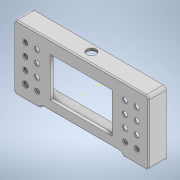
# Autodesk Inventor part: CONTROL_BOARD
Saved by Autodesk Inventor 2020 (Build 240168000, 168)
## iProperties
Created: 2020-06-05
Part Number: CONTROL_BOARD
Material: Generic
Document SubType Name: Modeling
Designer: Gebruiker
Density: 1 g/cm^3
Appearance: Default
Author: Gebruiker
Autodesk Inventor part; units mm, degrees
ref_plane "YZ Plane" through (0, 0, 0) normal (1, 0, 0) x (0, 1, 0)
ref_plane "XZ Plane" through (0, 0, 0) normal (0, 1, 0) x (-1, 0, 0)
ref_plane "XY Plane" through (0, 0, 0) normal (0, 0, 1) x (1, 0, 0)
sketch "Sketch1" plane through (0, 0, 0) normal (0, 0, 1) x (1, 0, 0)
  line L0 (-92.5, -50) -> (92.5, -50)
  line L1 (92.5, -50) -> (92.5, 50)
  line L2 (92.5, 50) -> (-92.5, 50)
  line L3 (-92.5, 50) -> (-92.5, -50)
  line L4 (-92.5, -50) -> (92.5, 50) construction
  line L5 (92.5, -50) -> (-92.5, 50) construction
  line L6 (70, 55) -> (115, 55)
  line L7 (115, 55) -> (115, 45)
  line L8 (115, 45) -> (70, 45)
  line L9 (70, 45) -> (70, 55)
  line L10 (70, 55) -> (115, 45) construction
  line L11 (115, 55) -> (70, 45) construction
  line L12 (70, -45) -> (115, -45)
  line L13 (115, -45) -> (115, -55)
  line L14 (115, -55) -> (70, -55)
  line L15 (70, -55) -> (70, -45)
  line L16 (70, -45) -> (115, -55) construction
  line L17 (115, -45) -> (70, -55) construction
  line L18 (-115, -45) -> (-70, -45)
  line L19 (-70, -45) -> (-70, -55)
  line L20 (-70, -55) -> (-115, -55)
  line L21 (-115, -55) -> (-115, -45)
  line L22 (-115, -45) -> (-70, -55) construction
  line L23 (-70, -45) -> (-115, -55) construction
  line L24 (-115, 55) -> (-70, 55)
  line L25 (-70, 55) -> (-70, 45)
  line L26 (-70, 45) -> (-115, 45)
  line L27 (-115, 45) -> (-115, 55)
  line L28 (-115, 55) -> (-70, 45) construction
  line L29 (-70, 55) -> (-115, 45) construction
  line L30 (70, 45) -> (115, 45)
  line L31 (115, 45) -> (115, -45)
  line L32 (115, -45) -> (70, -45)
  line L33 (70, -45) -> (70, 45)
  line L34 (70, 45) -> (115, -45) construction
  line L35 (115, 45) -> (70, -45) construction
  line L36 (-115, 45) -> (-70, 45)
  line L37 (-70, 45) -> (-70, -45)
  line L38 (-70, -45) -> (-115, -45)
  line L39 (-115, -45) -> (-115, 45)
  line L40 (-115, 45) -> (-70, -45) construction
  line L41 (-70, 45) -> (-115, -45) construction
  line L42 (115, 45) -> (115, 25)
  line L43 (115, -45) -> (115, -25)
  line L44 (-115, -45) -> (-115, -25)
  line L45 (-115, 45) -> (-115, 25)
  line L46 (-70, 55) -> (70, 55)
  line L47 (70, 55) -> (70, 50)
  line L48 (70, 50) -> (-70, 50)
  line L49 (-70, 50) -> (-70, 55)
  point P0 (0, 0)
  point P1 (92.5, 0)
  point P2 (-92.5, 0)
  point P3 (-70, -50)
  point P4 (70, -50)
  dimension "d0" = 185
  dimension "d1" = 100
  dimension "d2" = 45
  dimension "d3" = 10
  dimension "d4" = 45
  dimension "d5" = 10
  dimension "d6" = 45
  dimension "d7" = 45
  dimension "d8" = 10
  dimension "d9" = 45
  dimension "d10" = 90
  dimension "d20" = 20
  dimension "d21" = 20
  dimension "d22" = 20
  dimension "d23" = 20
  dimension "d83" = 45
  constraints: 100 end point, 17 midpoint, 16 parallel, 8 horizontal, 8 perpendicular, 6 point on line, 1 collinear
  measures "d0" distance of L2.end L1.end
  measures "d1" distance of L1.end L0.end
  measures "d2" distance of L7.end L8.end
  measures "d3" distance of L6.end L7.end
  measures "d4" distance of L13.end L14.end
  measures "d5" distance of L12.end L13.end
  measures "d6" distance of L19.end L20.end
  measures "d7" distance of L25.end L26.end
  measures "d8" distance of L24.end L25.end
  measures "d9" distance of L31.end L32.end
  measures "d10" distance of L36.end L37.end
  measures "d20" distance of L7.end L42.end
  measures "d21" distance of L12.end L43.end
  measures "d22" distance of L18.start L44.end
  measures "d23" distance of L26.end L45.end
  measures "d83" distance of L37.end L38.end
extrude "Extrusion1" add sketch "Sketch1" against normal blind 30
fillet "Fillet1" radius 5 8 edges at (-115, 55, -15) (-115, -55, -15) (-70, -55, -15) (-70, -50, -15) (70, -50, -15) (70, -55, -15) (115, -55, -15) (115, 55, -15)
sketch "Sketch5" plane through (0, 0, -30) normal (0, 0, -1) x (-1, 0, 0)
  line L0 (-109, 44) -> (109, 44)
  line L1 (109, 44) -> (109, -44)
  line L2 (109, -44) -> (-109, -44)
  line L3 (-109, -44) -> (-109, 44)
  line L4 (-109, 44) -> (109, -44) construction
  line L5 (109, 44) -> (-109, -44) construction
  point P0 (0, 0)
  dimension "d51" = 218
  dimension "d52" = 88
  constraints: 12 end point, 2 midpoint, 2 parallel, 1 horizontal, 1 perpendicular
  measures "d51" distance of L1.end L2.end
  measures "d52" distance of L0.end L1.end
extrude "Extrusion5" cut sketch "Sketch5" against normal blind 25
sketch "Sketch6" plane through (0, 0, 0) normal (0, 0, 1) x (1, 0, 0)
  line L0 (-53, 34) -> (53, 34)
  line L1 (53, 34) -> (53, -34)
  line L2 (53, -34) -> (-53, -34)
  line L3 (-53, -34) -> (-53, 34)
  line L4 (-53, 34) -> (53, -34) construction
  line L5 (53, 34) -> (-53, -34) construction
  point P0 (0, 0)
  dimension "d56" = 106
  dimension "d57" = 68
  constraints: 12 end point, 2 midpoint, 2 parallel, 1 horizontal, 1 perpendicular
  measures "d56" distance of L1.end L2.end
  measures "d57" distance of L0.end L1.end
extrude "Extrusion6" cut sketch "Sketch6" against normal blind 5
sketch "Sketch7" plane through (0, 0, 0) normal (0, 0, 1) x (1, 0, 0)
  line L0 (-53, -34) -> (-53, 34) projected
  line L1 (-53, 34) -> (53, 34) projected
  line L2 (53, 34) -> (53, -34) projected
  line L3 (53, -34) -> (-53, -34) projected
  arc A0 (-110, 55) -> (-115, 50) centre (-110, 50) ccw projected
  arc A1 (-115, -50) -> (-110, -55) centre (-110, -50) ccw projected
  line L4 (-110, -55) -> (-73.6603, -55) projected
  arc A2 (-73.6603, -55) -> (-69.3301, -52.5) centre (-73.6603, -50) ccw projected
  arc A3 (-65, -50) -> (-69.3301, -52.5) centre (-65, -55) ccw projected
  line L5 (-65, -50) -> (65, -50) projected
  arc A4 (69.3301, -52.5) -> (65, -50) centre (65, -55) ccw projected
  arc A5 (69.3301, -52.5) -> (73.6603, -55) centre (73.6603, -50) ccw projected
  line L6 (73.6603, -55) -> (110, -55) projected
  arc A6 (110, -55) -> (115, -50) centre (110, -50) ccw projected
  arc A7 (115, 50) -> (110, 55) centre (110, 50) ccw projected
  line L7 (110, 55) -> (-110, 55) projected
  line L8 (4.825, 59.0166) -> (4.825, -53.5355) construction
  line L9 (-115, 50) -> (-115, -50) projected
  line L10 (115, -50) -> (115, 50) projected
  point P0 (0, 0)
  constraints: 2 end point, 1 vertical
sketch "Sketch8" plane through (0, 0, 0) normal (0, 0, 1) x (1, 0, 0)
  line L0 (67.7, 39.3) -> (83, 39.3)
  line L1 (83, 39.3) -> (83, 24.3)
  line L2 (83, 24.3) -> (67.7, 24.3)
  line L3 (67.7, 24.3) -> (67.7, 39.3)
  line L4 (87.7, 39.3) -> (103, 39.3)
  line L5 (103, 39.3) -> (103, 24.3)
  line L6 (103, 24.3) -> (87.7, 24.3)
  line L7 (87.7, 24.3) -> (87.7, 39.3)
  line L8 (67.7, 16.5) -> (83, 16.5)
  line L9 (83, 16.5) -> (83, 4.2)
  line L10 (83, 4.2) -> (67.7, 4.2)
  line L11 (67.7, 4.2) -> (67.7, 16.5)
  line L12 (87.7, 16.5) -> (103, 16.5)
  line L13 (103, 16.5) -> (103, 4.2)
  line L14 (103, 4.2) -> (87.7, 4.2)
  line L15 (87.7, 4.2) -> (87.7, 16.5)
  line L16 (-123.4592, 0) -> (132.261, 0) construction
  line L17 (0, 57.3995) -> (0, -58.2893) construction
  line L18 (67.7, -39.3) -> (83, -39.3)
  line L19 (83, -39.3) -> (83, -24.3)
  line L20 (83, -24.3) -> (67.7, -24.3)
  line L21 (67.7, -24.3) -> (67.7, -39.3)
  line L22 (87.7, -39.3) -> (103, -39.3)
  line L23 (103, -39.3) -> (103, -24.3)
  line L24 (103, -24.3) -> (87.7, -24.3)
  line L25 (87.7, -24.3) -> (87.7, -39.3)
  line L26 (67.7, -16.5) -> (83, -16.5)
  line L27 (83, -16.5) -> (83, -4.2)
  line L28 (83, -4.2) -> (67.7, -4.2)
  line L29 (67.7, -4.2) -> (67.7, -16.5)
  line L30 (87.7, -16.5) -> (103, -16.5)
  line L31 (103, -16.5) -> (103, -4.2)
  line L32 (103, -4.2) -> (87.7, -4.2)
  line L33 (87.7, -4.2) -> (87.7, -16.5)
  line L34 (-67.7, 39.3) -> (-83, 39.3)
  line L35 (-83, 39.3) -> (-83, 24.3)
  line L36 (-83, 24.3) -> (-67.7, 24.3)
  line L37 (-67.7, 24.3) -> (-67.7, 39.3)
  line L38 (-87.7, 39.3) -> (-103, 39.3)
  line L39 (-103, 39.3) -> (-103, 24.3)
  line L40 (-103, 24.3) -> (-87.7, 24.3)
  line L41 (-87.7, 24.3) -> (-87.7, 39.3)
  line L42 (-67.7, 16.5) -> (-83, 16.5)
  line L43 (-83, 16.5) -> (-83, 4.2)
  line L44 (-83, 4.2) -> (-67.7, 4.2)
  line L45 (-67.7, 4.2) -> (-67.7, 16.5)
  line L46 (-87.7, 16.5) -> (-103, 16.5)
  line L47 (-103, 16.5) -> (-103, 4.2)
  line L48 (-103, 4.2) -> (-87.7, 4.2)
  line L49 (-87.7, 4.2) -> (-87.7, 16.5)
  line L50 (-67.7, -39.3) -> (-83, -39.3)
  line L51 (-67.7, -24.3) -> (-67.7, -39.3)
  line L52 (-83, -24.3) -> (-67.7, -24.3)
  line L53 (-83, -39.3) -> (-83, -24.3)
  line L54 (-87.7, -24.3) -> (-87.7, -39.3)
  line L55 (-103, -24.3) -> (-87.7, -24.3)
  line L56 (-103, -39.3) -> (-103, -24.3)
  line L57 (-87.7, -39.3) -> (-103, -39.3)
  line L58 (-67.7, -16.5) -> (-83, -16.5)
  line L59 (-67.7, -4.2) -> (-67.7, -16.5)
  line L60 (-83, -4.2) -> (-67.7, -4.2)
  line L61 (-83, -16.5) -> (-83, -4.2)
  line L62 (-87.7, -4.2) -> (-87.7, -16.5)
  line L63 (-87.7, -16.5) -> (-103, -16.5)
  line L64 (-103, -16.5) -> (-103, -4.2)
  line L65 (-103, -4.2) -> (-87.7, -4.2)
  line L66 (-174.6033, 0) -> (183.4051, 0) projected
  line L67 (115, -50) -> (115, 50) projected
  line L68 (-115, 50) -> (-115, -50) projected
  line L69 (75.35, 39.3) -> (75.35, 24.3) construction
  line L70 (95.35, 39.3) -> (95.35, 24.3) construction
  line L71 (67.7, 24.3) -> (103, 24.3)
  line L72 (103, 24.3) -> (103, 16.5)
  line L73 (103, 16.5) -> (67.7, 16.5)
  line L74 (67.7, 16.5) -> (67.7, 24.3)
  line L75 (83, 39.3) -> (87.7, 39.3)
  line L76 (87.7, 39.3) -> (87.7, 4.2)
  line L77 (87.7, 4.2) -> (83, 4.2)
  line L78 (83, 4.2) -> (83, 39.3)
  line L79 (67.7, 4.2) -> (103, 4.2)
  line L80 (103, 4.2) -> (103, -4.2)
  line L81 (103, -4.2) -> (67.7, -4.2)
  line L82 (67.7, -4.2) -> (67.7, 4.2)
  line L83 (83, -39.3) -> (83, -24.3)
  line L84 (83, -24.3) -> (67.7, -24.3)
  line L85 (103, -24.3) -> (87.7, -24.3)
  line L86 (87.7, -24.3) -> (87.7, -39.3)
  line L87 (67.7, -16.5) -> (83, -16.5)
  line L88 (83, -4.2) -> (67.7, -4.2)
  line L89 (87.7, -16.5) -> (103, -16.5)
  line L90 (103, -4.2) -> (87.7, -4.2)
  line L91 (103, -24.3) -> (103, -16.5)
  line L92 (67.7, -16.5) -> (67.7, -24.3)
  line L93 (83, -39.3) -> (87.7, -39.3)
  line L94 (87.7, -39.3) -> (87.7, -4.2)
  line L95 (87.7, -4.2) -> (83, -4.2)
  line L96 (83, -4.2) -> (83, -39.3)
  line L97 (103, -4.2) -> (103, 4.2)
  line L98 (67.7, 4.2) -> (67.7, -4.2)
  line L99 (-83, 39.3) -> (-83, 24.3)
  line L100 (-103, 24.3) -> (-87.7, 24.3)
  line L101 (-87.7, 24.3) -> (-87.7, 39.3)
  line L102 (-67.7, 16.5) -> (-83, 16.5)
  line L103 (-83, 16.5) -> (-83, 4.2)
  line L104 (-87.7, 16.5) -> (-103, 16.5)
  line L105 (-87.7, 4.2) -> (-87.7, 16.5)
  line L106 (-83, -24.3) -> (-67.7, -24.3)
  line L107 (-103, -24.3) -> (-87.7, -24.3)
  line L108 (-67.7, -16.5) -> (-83, -16.5)
  line L109 (-87.7, -16.5) -> (-103, -16.5)
  line L110 (-103, 24.3) -> (-103, 16.5)
  line L111 (-67.7, 16.5) -> (-67.7, 24.3)
  line L112 (-83, 39.3) -> (-87.7, 39.3)
  line L113 (-67.7, 4.2) -> (-103, 4.2)
  line L114 (-103, 4.2) -> (-103, -4.2)
  line L115 (-103, -4.2) -> (-67.7, -4.2)
  line L116 (-67.7, -4.2) -> (-67.7, 4.2)
  line L117 (-83, -39.3) -> (-87.7, -39.3)
  line L118 (-87.7, -39.3) -> (-87.7, -4.2)
  line L119 (-83, -4.2) -> (-83, -39.3)
  line L120 (-67.7, -16.5) -> (-67.7, -24.3)
  line L121 (-103, -24.3) -> (-103, -16.5)
  line L122 (103, -39.3) -> (105, -39.3)
  line L123 (105, -39.3) -> (105, 39.3)
  line L124 (105, 39.3) -> (103, 39.3)
  line L125 (103, 39.3) -> (103, -39.3)
  line L126 (67.7, -39.3) -> (66.7, -39.3)
  line L127 (66.7, -39.3) -> (66.7, 39.3)
  line L128 (66.7, 39.3) -> (67.7, 39.3)
  line L129 (67.7, 39.3) -> (67.7, -39.3)
  line L130 (-67.7, -39.3) -> (-66.7, -39.3)
  line L131 (-66.7, -39.3) -> (-66.7, 39.3)
  line L132 (-66.7, 39.3) -> (-67.7, 39.3)
  line L133 (-67.7, 39.3) -> (-67.7, -39.3)
  line L134 (-103, -39.3) -> (-105, -39.3)
  line L135 (-105, -39.3) -> (-105, 39.3)
  line L136 (-105, 39.3) -> (-103, 39.3)
  line L137 (-103, 39.3) -> (-103, -39.3)
  point P0 (0, 0)
  point P1 (83, 4.2)
  point P2 (-75.35, 24.3)
  point P3 (83, 4.2)
  dimension "d106" = 15.3
  dimension "d107" = 15
  dimension "d108" = 15.3
  dimension "d109" = 12.3
  dimension "d110" = 7.8
  dimension "d112" = 4.2
  dimension "d113" = 12
  dimension "d115" = 12
  dimension "d128" = 20
  dimension "d184" = 7.8
  dimension "d213" = 2
  dimension "d214" = 1
  dimension "d215" = 1
  dimension "d216" = 2
  constraints: 270 end point, 79 symmetric about line, 44 point on line, 22 parallel, 12 horizontal, 11 perpendicular, 4 midpoint, 1 collinear, 1 vertical
  measures "d106" distance of L1.end L2.end
  measures "d107" distance of L0.end L1.end
  measures "d108" distance of L5.end L6.end
  measures "d109" distance of L8.end L9.end
  measures "d110" distance between parallel lines of L12 L6
  measures "d112" distance between parallel lines of L16 L14
  measures "d113" distance between parallel lines of L67 L5
  measures "d115" distance between parallel lines of L68 L39
  measures "d128" distance between parallel lines of L70 L69
  measures "d184" distance between parallel lines of L24 L30
  measures "d213" distance of L124.end L123.end
  measures "d214" distance of L127.end L128.end
  measures "d215" distance of L132.end L131.end
  measures "d216" distance of L135.end L136.end
extrude "Extrusion10" cut sketch "Sketch8" against normal blind 5
sketch "Sketch13" plane through (0, 0, -30) normal (0, 0, -1) x (-1, 0, 0)
  line L0 (-109, 44) -> (109, 44) projected
  line L1 (101, 44) -> (80.8, 44)
  line L2 (80.8, 44) -> (80.8, 52.2)
  line L3 (80.8, 52.2) -> (101, 52.2)
  line L4 (101, 52.2) -> (101, 44)
  line L5 (115, -50) -> (115, 50) projected
  point P0 (0, 0)
  dimension "d151" = 20.2
  dimension "d152" = 8.2
  dimension "d153" = 14
  constraints: 8 end point, 2 parallel, 1 horizontal, 1 perpendicular, 1 point on line
  measures "d151" distance of L2.end L3.end
  measures "d152" distance of L1.end L2.end
  measures "d153" distance between parallel lines of L5 L4
extrude "Extrusion16" cut sketch "Sketch13" against normal blind 5
mirror "Mirror3" about plane through (0, 0, 0) normal (1, 0, 0) of "Extrusion16"
sketch "Sketch17" plane through (0, 0, -5) normal (0, 0, -1) x (-1, 0, 0)
  circle A0 centre (102.9761, 38.9853) radius 1.5 projected
  circle A1 centre (65.4761, 38.9853) radius 1.5 projected
  circle A2 centre (102.9761, -38.5147) radius 1.5 projected
  circle A3 centre (65.4761, -38.5147) radius 1.5 projected
  circle A4 centre (56.7761, -33.5647) radius 1.6 projected
  circle A5 centre (56.7761, 33.9353) radius 1.6 projected
  circle A6 centre (-56.7239, 33.9353) radius 1.6 projected
  circle A7 centre (-56.7239, -33.5647) radius 1.6 projected
  line L0 (-53, 34) -> (53, 34) projected
  line L1 (53, 34) -> (53, -34) projected
  line L2 (53, -34) -> (-53, -34) projected
  line L3 (-53, -34) -> (-53, 34) projected
  line L4 (-109, 44) -> (109, 44) projected
  line L5 (-109, -44) -> (-109, 44) projected
  line L6 (109, -44) -> (-109, -44) projected
  line L7 (109, 44) -> (109, -44) projected
  circle A8 centre (-65.4239, -38.5147) radius 1.5 projected
  circle A9 centre (-102.9239, -38.5147) radius 1.5 projected
  circle A10 centre (-102.9239, 38.9853) radius 1.5 projected
  circle A11 centre (-65.4239, 38.9853) radius 1.5 projected
  point P0 (0, 0)
hole "Hole1" at (-102.9761, 38.9853, -5) at (-102.9761, -38.5147, -5) at (-65.4761, -38.5147, -5) at (-56.7761, -33.5647, -5) at (-65.4761, 38.9853, -5) at (-56.7761, 33.9353, -5) at (56.7239, -33.5647, -5) at (56.7239, 33.9353, -5) at (65.4239, 38.9853, -5) at (102.9239, 38.9853, -5) at (102.9239, -38.5147, -5) at (65.4239, -38.5147, -5) direction (0, 0, 1) diameter 2.459 depth 2 tip angle 118 thread size "M3x0.5" class "6H" standard "ISO Metric profile"
sketch "Sketch18" plane through (0, 0, -30) normal (0, 0, -1) x (-1, 0, 0)
  point P0 (0, 0)
sketch "Sketch19" plane through (0, 0, -30) normal (0, 0, -1) x (-1, 0, 0)
  circle A0 centre (108, 48) radius 2.25 projected
  circle A1 centre (108, -48) radius 2.25 projected
  circle A2 centre (-108, -48) radius 2.25 projected
  circle A3 centre (-108, 48) radius 2.25 projected
  point P0 (0, 0)
hole "Hole2" at (-108, 48, -30) at (-108, -48, -30) at (108, -48, -30) at (108, 48, -30) direction (0, 0, 1) diameter 2.459 depth 5 tip angle 118 thread size "M3x0.5" class "6H" standard "ISO Metric profile"
fillet "Fillet6" radius 2 14 edges at (-113.5355, 53.5355, 0) (-115, 0, 0) (-113.5355, -53.5355, 0) (-91.8301, -55, 0) (-71.1603, -54.3301, 0) (-67.5001, -50.6699, 0) (0, -50, 0) (67.5001, -50.6699, 0) (71.1603, -54.3301, 0) (91.8301, -55, 0) (113.5355, -53.5355, 0) (115, 0, 0) (113.5355, 53.5355, 0) (0, 55, 0)
sketch "Sketch20" plane through (0, 0, -30) normal (0, 0, -1) x (-1, 0, 0)
  line L0 (-52.5, 51) -> (52.5, 51)
  line L1 (52.5, 51) -> (52.5, 37)
  line L2 (52.5, 37) -> (-52.5, 37)
  line L3 (-52.5, 37) -> (-52.5, 51)
  line L4 (-80.8, 44) -> (80.8, 44) projected
  line L5 (-52.5, 51) -> (52.5, 37) construction
  line L6 (52.5, 51) -> (-52.5, 37) construction
  point P0 (0, 0)
  point P1 (0, 44)
  point P2 (-52.5, 44)
  point P3 (52.5, 44)
  dimension "d180" = 105
  dimension "d181" = 14
  constraints: 12 end point, 3 midpoint, 2 parallel, 1 horizontal, 1 perpendicular
  measures "d180" distance of L1.end L2.end
  measures "d181" distance of L0.end L1.end
extrude "Extrusion20" cut sketch "Sketch20" against normal blind 25 contours L0 L1 L4 L3
sketch "Sketch21" plane through (-110, 55, -30) normal (0, 1, 0) x (1, 0, 0)
  line L0 (57, -25) -> (163, -25) construction
  line L1 (110, -25) -> (110, 0) construction
  line L2 (162.5, 0) -> (57.5, 0) construction
  circle A0 centre (110, -12.5) radius 8
  point P0 (110, -30)
  dimension "d185" = 16
  constraints: 3 midpoint, 2 end point, 1 centre point
  measures "d185" diameter of A0
extrude "Extrusion21" cut sketch "Sketch21" against normal blind 5
sketch "Sketch22" plane through (0, 0, 0) normal (0, 0, 1) x (1, 0, 0)
  circle A0 centre (-95, 30) radius 4.25
  line L0 (110, 55) -> (-110, 55) projected
  line L1 (-115, 50) -> (-115, -50) projected
  circle A1 centre (-75, 30) radius 4.25
  circle A2 centre (-95, 9.4) radius 4.25
  circle A3 centre (-75, 9.4) radius 4.25
  line L2 (-122.9907, -0.9) -> (134.9522, -0.9) construction
  line L3 (-67.7, 39.3) -> (-101.7876, 39.3) construction
  line L4 (-84.7438, 39.3) -> (-84.7438, -0.9) construction
  circle A4 centre (-95, -31.8) radius 4.25
  circle A5 centre (-75, -31.8) radius 4.25
  circle A6 centre (-95, -11.2) radius 4.25
  circle A7 centre (-75, -11.2) radius 4.25
  line L5 (0, 62.7559) -> (0, -64.4436) construction
  circle A8 centre (95, 30) radius 4.25
  circle A9 centre (75, 30) radius 4.25
  circle A10 centre (95, 9.4) radius 4.25
  circle A11 centre (75, 9.4) radius 4.25
  circle A12 centre (95, -31.8) radius 4.25
  circle A13 centre (75, -31.8) radius 4.25
  circle A14 centre (95, -11.2) radius 4.25
  circle A15 centre (75, -11.2) radius 4.25
  line L6 (-110, -55) -> (-73.6603, -55) construction
  point P0 (0, 0)
  dimension "d194" = 8.5
  dimension "d195" = 25
  dimension "d196" = 20
  dimension "d197" = 8.5
  dimension "d198" = 25
  dimension "d199" = 20
  dimension "d200" = 8.5
  dimension "d201" = 20
  dimension "d202" = 20.6
  dimension "d203" = 8.5
  dimension "d204" = 20.6
  dimension "d205" = 20
  dimension "d206" = 20.6
  dimension "d207" = 23.2
  constraints: 16 centre point, 12 symmetric about line, 6 end point, 1 horizontal, 1 midpoint, 1 perpendicular, 1 point on line, 1 vertical, 12 other
  measures "d194" diameter of A0
  measures "d195" distance from line of A0.centre L0
  measures "d196" distance from line of L1 A0.centre
  measures "d197" diameter of A1
  measures "d198" distance from line of A1.centre L0
  measures "d199" distance of A1.centre A0.centre
  measures "d200" diameter of A2
  measures "d201" distance from line of L1 A2.centre
  measures "d202" distance of A2.centre A0.centre
  measures "d203" diameter of A3
  measures "d204" distance of A3.centre A1.centre
  measures "d205" distance of A2.centre A3.centre
  measures "d206" distance of A6.centre A2.centre
  measures "d207" distance from line of L6 A4.centre
sketch "Sketch23" plane through (0, 0, 0) normal (0, 0, 1) x (1, 0, 0)
  point P0 (0, 0)
sketch "Sketch24" plane through (0, 0, 0) normal (0, 0, 1) x (1, 0, 0)
  circle A0 centre (-95, 30) radius 4.25 projected
  circle A1 centre (-75, 30) radius 4.25 projected
  circle A2 centre (-95, 9.4) radius 4.25 projected
  circle A3 centre (-75, 9.4) radius 4.25 projected
  circle A4 centre (-95, -11.2) radius 4.25 projected
  circle A5 centre (-75, -11.2) radius 4.25 projected
  circle A6 centre (-95, -31.8) radius 4.25 projected
  circle A7 centre (-75, -31.8) radius 4.25 projected
  circle A8 centre (75, 30) radius 4.25 projected
  circle A9 centre (95, 30) radius 4.25 projected
  circle A10 centre (75, 9.4) radius 4.25 projected
  circle A11 centre (95, 9.4) radius 4.25 projected
  circle A12 centre (75, -11.2) radius 4.25 projected
  circle A13 centre (95, -11.2) radius 4.25 projected
  circle A14 centre (75, -31.8) radius 4.25 projected
  circle A15 centre (95, -31.8) radius 4.25 projected
  line L0 (-105.0659, 39.3) -> (-66.7, 39.3)
  line L1 (-66.7, -39.3) -> (-105.0659, -39.3)
  line L2 (-105.0659, -39.3) -> (-105.0659, 39.3)
  line L3 (-102.0301, -39.3) -> (-66.7, -39.3) projected
  line L4 (-66.7, 39.3) -> (-66.7, -39.3)
  line L5 (105, -39.3) -> (105, 39.3) projected
  line L6 (66.6788, 39.3) -> (105, 39.3)
  line L7 (105, 39.3) -> (105, -39.3)
  line L8 (105, -39.3) -> (66.6788, -39.3)
  line L9 (66.6788, -39.3) -> (66.6788, 39.3)
  point P0 (0, 0)
  point P1 (67.7, 39.3)
  point P2 (103, -39.3)
  constraints: 16 end point, 3 parallel, 2 horizontal, 2 perpendicular
extrude "Extrusion22" add sketch "Sketch24" against normal blind 2
sketch "Sketch25" plane through (0, 0, 0) normal (0, 0, 1) x (1, 0, 0)
  circle A0 centre (-95, -31.8) radius 4.25 projected
  circle A1 centre (-95, -31.8) radius 5
  point P0 (0, 0)
  dimension "d210" = 10
  constraints: 1 centre point, 1 coincident
  measures "d210" diameter of A1
extrude "Extrusion23" cut sketch "Sketch25" against normal blind 2
body "Solid1"
